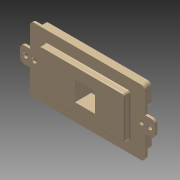
# Autodesk Inventor part: Wall_Switch_June_8_2017_Front._Sppt
Saved by Autodesk Inventor 2015 (Build 190159000, 159)
## iProperties
Created: 2014-05-05
Part Number: Wall_Switch_June_8_2017_Front._Sppt
Material: ABS Plastic
Document SubType Name: Modeling
Designer: admin
Density: 1.06 g/cm^3
Appearance: Smooth - Off-White
Author: admin
Autodesk Inventor part; units mm, degrees
sketch "Sketch1" plane through (0, 0, 0) normal (0, 0, 1) x (1, 0, 0)
  line L0 (-46.99, 28.575) -> (46.99, 28.575)
  line L1 (46.99, 28.575) -> (46.99, -28.575)
  line L2 (46.99, -28.575) -> (-46.99, -28.575)
  line L3 (-46.99, -28.575) -> (-46.99, 28.575)
  line L4 (45.2735, 26.416) -> (-44.3885, 26.416)
  line L5 (-44.831, -26.416) -> (44.831, -26.416)
  circle A0 centre (41.656, 0) radius 1.5875
  circle A1 centre (-41.656, -0.0059) radius 1.5875
  arc A2 (41.656, 3.175) -> (41.656, -3.175) centre (41.656, 0) ccw
  line L6 (-41.656, 3.1691) -> (-44.3885, 3.1691)
  line L7 (-41.656, -3.1809) -> (-44.831, -3.1809)
  line L8 (41.656, -3.175) -> (44.831, -3.175)
  line L9 (41.656, 3.175) -> (45.2735, 3.175)
  line L10 (44.831, -26.416) -> (44.831, -3.175)
  line L11 (45.2735, 3.175) -> (45.2735, 26.416)
  line L12 (-44.3885, 26.416) -> (-44.3885, 3.1691)
  arc A3 (-41.656, -3.1809) -> (-41.656, 3.1691) centre (-41.656, -0.0059) ccw
  line L13 (-44.831, -3.1809) -> (-44.831, -26.416)
  point P0 (0, 0)
  point P1 (0, 28.575)
  point P2 (-46.99, 0)
  constraints: 28 end point, 11 perpendicular, 7 parallel, 4 centre point, 4 point on circle, 4 tangent, 2 midpoint, 1 horizontal, 1 horizontal alignment, 1 vertical alignment
ref_plane "Work Plane1" through (0, 0, 0) normal (0, 0, 1) x (1, 0, 0)
sketch "Sketch2" plane through (0, 0, 0) normal (0, 0, 1) x (1, 0, 0)
  circle A0 centre (-41.656, -0.0059) radius 1.5875 projected
  circle A1 centre (41.656, 0) radius 1.5875 projected
  line L0 (-52.451, 25.4) -> (52.451, 25.4)
  line L1 (52.451, 25.4) -> (52.451, -25.4)
  line L2 (52.451, -25.4) -> (-52.451, -25.4)
  line L3 (-52.451, -25.4) -> (-52.451, 25.4)
  circle A2 centre (-41.656, -0.0059) radius 1.5875
  circle A3 centre (41.656, 0) radius 1.5875
  point P0 (0, 0)
  point P1 (0, 25.4)
  point P2 (52.451, 0)
  point P3 (-41.656, 0)
  point P4 (0, 12.7)
  dimension "d10" = 104.902
  dimension "d11" = 50.8
  constraints: 8 end point, 2 centre point, 2 coincident, 2 horizontal alignment, 2 midpoint, 2 parallel, 2 vertical alignment, 1 horizontal, 1 perpendicular
  measures "d10" distance of L1.end L2.end
  measures "d11" distance of L0.end L1.end
extrude "Extrusion2" add sketch "Sketch2" along normal blind 1.905
ref_plane "Work Plane3" through (0, 0, 2.54) normal (0, 0, 1) x (1, 0, 0)
sketch "Sketch4" plane through (0, 0, 2.54) normal (0, 0, 1) x (1, 0, 0)
  line L0 (-33.0835, 16.383) -> (33.0835, 16.383)
  line L1 (33.0835, 16.383) -> (33.0835, -16.383)
  line L2 (33.0835, -16.383) -> (-33.0835, -16.383)
  line L3 (-33.0835, -16.383) -> (-33.0835, 16.383)
  point P0 (0, 0)
  point P1 (0, 16.383)
  point P2 (33.0835, 0)
  dimension "d22" = 66.167
  dimension "d23" = 32.766
  constraints: 8 end point, 2 midpoint, 2 parallel, 1 horizontal, 1 horizontal alignment, 1 perpendicular, 1 vertical alignment
  measures "d22" distance of L1.end L2.end
  measures "d23" distance of L0.end L1.end
ref_plane "Work Plane2" through (0, 0, 0) normal (0, 0, -1) x (-1, 0, 0)
sketch "Sketch5" plane through (0, 0, 0) normal (0, 0, -1) x (-1, 0, 0)
  line L0 (44.3885, 3.1691) -> (44.3885, 25.4) projected
  line L1 (-45.2735, 25.4) -> (-45.2735, 3.175) projected
  line L2 (-45.2735, 3.175) -> (-41.656, 3.175) projected
  arc A0 (-41.656, -3.175) -> (-41.656, 3.175) centre (-41.656, 0) ccw projected
  line L3 (-41.656, -3.175) -> (-44.831, -3.175) projected
  line L4 (-44.831, -3.175) -> (-44.831, -25.4) projected
  line L5 (44.831, -25.4) -> (44.831, -3.1809) projected
  line L6 (44.831, -3.1809) -> (41.656, -3.1809) projected
  arc A1 (41.656, 3.1691) -> (41.656, -3.1809) centre (41.656, -0.0059) ccw projected
  line L7 (41.656, 3.1691) -> (44.3885, 3.1691) projected
  circle A2 centre (39.116, 12.7) radius 1.27
  circle A3 centre (39.116, -12.7) radius 1.27
  circle A4 centre (-39.116, -12.7) radius 1.27
  circle A5 centre (-39.116, 12.7) radius 1.27
  line L8 (-35.56, 20.32) -> (35.56, 20.32)
  line L9 (35.56, 20.32) -> (35.56, -20.32)
  line L10 (35.56, -20.32) -> (-35.56, -20.32)
  line L11 (-35.56, -20.32) -> (-35.56, 20.32)
  line L12 (46.99, -28.575) -> (46.99, 28.575) projected
  line L13 (-46.99, 28.575) -> (-46.99, -28.575) projected
  line L14 (-41.656, 22.86) -> (41.656, 22.86)
  line L15 (41.656, -22.86) -> (-41.656, -22.86)
  line L16 (-37.6174, 5.6991) -> (-37.6174, -5.6991)
  line L17 (37.6174, 5.6933) -> (37.6174, -5.705)
  arc A6 (37.6174, -5.705) -> (41.656, -6.9909) centre (41.656, -0.0059) ccw
  arc A7 (41.656, 6.9791) -> (37.6174, 5.6933) centre (41.656, -0.0059) ccw
  line L18 (41.656, 22.86) -> (41.656, 6.9791)
  line L19 (41.656, -6.9909) -> (41.656, -22.86)
  arc A8 (-37.6174, 5.6991) -> (-41.656, 6.985) centre (-41.656, 0) ccw
  arc A9 (-41.656, -6.985) -> (-37.6174, -5.6991) centre (-41.656, 0) ccw
  line L20 (-41.656, -22.86) -> (-41.656, -6.985)
  line L21 (-41.656, 6.985) -> (-41.656, 22.86)
  point P0 (0, 0)
  point P1 (-38.1, 0)
  point P2 (-35.56, 0)
  point P3 (0, 20.32)
  point P4 (0, 12.7)
  point P5 (41.656, -0.0059)
  dimension "d30" = 2.54
  dimension "d31" = 2.54
  dimension "d32" = 2.54
  dimension "d33" = 2.54
  dimension "d36" = 71.12
  dimension "d37" = 40.64
  dimension "d91" = 83.312
  dimension "d92" = 45.72
  dimension "d95" = 2.0574
  dimension "d205" = 2.54
  constraints: 26 end point, 10 parallel, 8 centre point, 8 point on circle, 4 vertical alignment, 3 coincident, 3 perpendicular, 2 horizontal, 2 horizontal alignment, 2 midpoint, 1 point on line
  measures "d30" diameter of A2
  measures "d31" diameter of A3
  measures "d32" diameter of A4
  measures "d33" diameter of A5
  measures "d36" distance of L9.end L10.end
  measures "d37" distance of L8.end L9.end
  measures "d91" distance of L15.start L15.end
  measures "d92" distance of L14.end L15.start
  measures "d95" distance between parallel lines of L17 L9
  measures "d205" distance between parallel lines of L8 L14
extrude "Extrusion8" add sketch "Sketch5" along normal blind 6.35
sketch "Sketch10" plane through (0, 0, 0) normal (0, 0, -1) x (-1, 0, 0)
  point P0 (0, 0)
sketch "Sketch7" plane through (0, 0, 0) normal (0, 0, -1) x (-1, 0, 0)
  line L0 (-33.02, 16.51) -> (33.02, 16.51)
  line L1 (33.02, 16.51) -> (33.02, -16.51)
  line L2 (33.02, -16.51) -> (-33.02, -16.51)
  line L3 (-33.02, -16.51) -> (-33.02, 16.51)
  point P0 (0, 0)
  point P1 (0, 16.51)
  point P2 (-33.02, 0)
  dimension "d55" = 66.04
  dimension "d56" = 33.02
  constraints: 8 end point, 2 midpoint, 2 parallel, 1 horizontal, 1 horizontal alignment, 1 perpendicular, 1 vertical alignment
  measures "d55" distance of L1.end L2.end
  measures "d56" distance of L0.end L1.end
sketch "Sketch8" plane through (0, 0, 1.905) normal (0, 0, 1) x (1, 0, 0)
  circle A0 centre (41.656, 0) radius 1.5875 projected
  circle A1 centre (-41.656, -0.0059) radius 1.5875 projected
  circle A2 centre (41.656, 0) radius 1.905
  circle A3 centre (-41.656, -0.0059) radius 1.905
  circle A4 centre (-48.387, 0) radius 1.905
  circle A5 centre (48.387, 0) radius 1.905
  point P0 (0, 0)
  dimension "d68" = 3.81
  dimension "d69" = 3.81
  dimension "d72" = 3.81
  dimension "d73" = 6.731
  dimension "d74" = 3.81
  dimension "d75" = 6.731
  constraints: 4 centre point, 2 coincident
  measures "d68" diameter of A2
  measures "d69" diameter of A3
  measures "d72" diameter of A4
  measures "d73" distance of A1.centre A4.centre
  measures "d74" diameter of A5
  measures "d75" distance of A5.centre A0.centre
extrude "Extrusion6" cut sketch "Sketch8" against normal blind 5.08
sketch "Sketch9" plane through (0, 0, 1.905) normal (0, 0, 1) x (1, 0, 0)
  line L0 (-52.451, 25.4) -> (-44.831, 25.4)
  line L1 (-44.831, 25.4) -> (-44.831, 6.35)
  line L2 (-44.831, 6.35) -> (-52.451, 6.35)
  line L3 (-52.451, 6.35) -> (-52.451, 25.4)
  line L4 (52.451, 25.4) -> (44.831, 25.4)
  line L5 (44.831, 25.4) -> (44.831, 6.35)
  line L6 (44.831, 6.35) -> (52.451, 6.35)
  line L7 (52.451, 6.35) -> (52.451, 25.4)
  line L8 (52.451, -25.4) -> (44.831, -25.4)
  line L9 (44.831, -25.4) -> (44.831, -6.35)
  line L10 (44.831, -6.35) -> (52.451, -6.35)
  line L11 (52.451, -6.35) -> (52.451, -25.4)
  line L12 (-52.451, -25.4) -> (-44.831, -25.4)
  line L13 (-44.831, -25.4) -> (-44.831, -6.35)
  line L14 (-44.831, -6.35) -> (-52.451, -6.35)
  line L15 (-52.451, -6.35) -> (-52.451, -25.4)
  line L16 (52.451, -25.4) -> (52.451, 25.4) projected
  point P0 (0, 0)
  point P1 (52.451, 15.875)
  point P2 (52.451, 0)
  dimension "d76" = 7.62
  dimension "d77" = 19.05
  dimension "d80" = 7.62
  dimension "d81" = 19.05
  dimension "d82" = 7.62
  dimension "d83" = 19.05
  dimension "d117" = 19.05
  dimension "d149" = 7.62
  constraints: 32 end point, 8 parallel, 4 horizontal, 4 perpendicular, 2 midpoint, 1 vertical alignment
  measures "d76" distance of L1.end L2.end
  measures "d77" distance of L0.end L1.end
  measures "d80" distance of L9.end L10.end
  measures "d81" distance of L8.end L9.end
  measures "d82" distance of L14.end L13.end
  measures "d83" distance of L13.end L12.end
  measures "d117" distance between parallel lines of L6 L4
  measures "d149" distance between parallel lines of L7 L5
extrude "Extrusion7" cut sketch "Sketch9" against normal blind 5.08
fillet "Fillet5" radius 3.175 8 edges at (44.831, 25.4, 0.9525) (52.451, 6.35, 0.9525) (-44.831, 25.4, 0.9525) (-52.451, 6.35, 0.9525) (52.451, -6.35, 0.9525) (44.831, -25.4, 0.9525) (-44.831, -25.4, 0.9525) (-52.451, -6.35, 0.9525)
fillet "Fillet7" radius 3.175 4 edges at (-41.656, -22.86, -3.175) (-41.656, 22.86, -3.175) (41.656, 22.86, -3.175) (41.656, -22.86, -3.175)
fillet "Fillet8" radius 3.175 4 edges at (-41.656, 6.9791, -3.175) (-41.656, -6.9909, -3.175) (41.656, 6.985, -3.175) (41.656, -6.985, -3.175)
sketch "Sketch13" plane through (0, 0, -6.35) normal (0, 0, -1) x (-1, 0, 0)
  line L0 (37.6174, -5.705) -> (37.6174, 5.6933) projected
  arc A0 (39.4732, 6.6293) -> (37.6174, 5.6933) centre (41.656, -0.0059) ccw projected
  line L1 (-37.6174, 5.6991) -> (-37.6174, -5.6991) projected
  arc A1 (-39.4732, -6.6352) -> (-37.6174, -5.6991) centre (-41.656, 0) ccw projected
  arc A2 (-37.6174, -3.0816) -> (-37.6174, 3.0816) centre (-41.656, 0) ccw
  arc A3 (37.6174, 3.0757) -> (37.6174, -3.0874) centre (41.656, -0.0059) ccw
  line L2 (37.6174, -3.0874) -> (37.6174, 3.0757)
  line L3 (-37.6174, -3.0816) -> (-37.6174, 3.0816)
  point P0 (0, 0)
  dimension "d107" = 10.16
  dimension "d108" = 10.16
  constraints: 4 end point, 4 point on circle, 4 point on line, 2 centre point, 2 coincident, 2 collinear
  measures "d107" diameter of A2
  measures "d108" diameter of A3
extrude "Extrusion9" [suppressed]
fillet "Fillet11" [suppressed]
fillet "Fillet12" [suppressed]
extrude "Extrusion17" add sketch "Sketch7" against normal blind 6.35
sketch "Sketch22" plane through (0, 0, 0) normal (0, 0, -1) x (-1, 0, 0)
  line L0 (-10.16, -7.7495) -> (5.3391, -7.7495)
  line L1 (5.3391, -7.7495) -> (5.3391, 7.7495)
  line L2 (5.3391, 7.7495) -> (-10.16, 7.7495)
  line L3 (-10.16, 7.7495) -> (-10.16, -7.7495)
  line L4 (-33.02, 16.51) -> (-33.02, -16.51) projected
  line L5 (41.656, 9.6453) -> (41.656, 19.685) projected
  point P0 (0, 0)
  point P1 (-33.02, 15.875)
  point P2 (-33.02, -15.875)
  point P3 (-10.16, 0)
  dimension "d194" = 15.4991
  dimension "d195" = 15.4991
  dimension "d197" = 51.816
  constraints: 8 end point, 2 parallel, 1 horizontal, 1 horizontal alignment, 1 midpoint, 1 perpendicular
  measures "d194" distance of L2.end L0.start
  measures "d195" distance of L1.end L2.end
  measures "d197" distance between parallel lines of L3 L5
extrude "Extrusion18" cut sketch "Sketch22" against normal blind 25.4
sketch "Sketch23" plane through (0, 0, 0) normal (0, 0, -1) x (-1, 0, 0)
  line L0 (5.3391, 7.7495) -> (-10.16, 7.7495)
  line L1 (-10.16, 7.7495) -> (-10.16, -7.7495)
  line L2 (-10.16, -7.7495) -> (5.3391, -7.7495)
  line L3 (5.3391, -7.7495) -> (5.3391, 7.7495)
  line L4 (-11.684, 9.2735) -> (6.8631, 9.2735)
  line L5 (6.8631, 9.2735) -> (6.8631, -9.2735)
  line L6 (6.8631, -9.2735) -> (-11.684, -9.2735)
  line L7 (-11.684, -9.2735) -> (-11.684, 9.2735)
  point P0 (0, 0)
  dimension "d201" = 1.524
  constraints: 16 end point, 4 parallel, 2 perpendicular, 1 horizontal, 3 other
  measures "d201" distance between parallel lines of L0 L4
extrude "Extrusion19" add sketch "Sketch23" along normal blind 6.35
fillet "Fillet17" radius 1.27 4 edges at (11.684, 9.2735, -3.175) (-6.8631, 9.2735, -3.175) (11.684, -9.2735, -3.175) (-6.8631, -9.2735, -3.175)
fillet "Fillet20" radius 1.905 4 edges at (-33.02, -16.51, 4.1275) (-33.02, 16.51, 4.1275) (33.02, -16.51, 4.1275) (33.02, 16.51, 4.1275)
sketch "Sketch24" plane through (0, 0, -6.35) normal (0, 0, -1) x (-1, 0, 0)
  circle A0 centre (37.5285, 18.7325) radius 1.5875
  line L0 (-35.56, 20.32) -> (35.56, 20.32)
  line L1 (35.56, 20.32) -> (35.56, -20.32)
  line L2 (35.56, -20.32) -> (-35.56, -20.32)
  line L3 (-35.56, -20.32) -> (-35.56, 20.32)
  line L4 (35.56, -20.32) -> (35.56, 20.32) projected
  line L5 (38.0025, 17.2174) -> (43.4689, 17.2174) construction
  line L6 (41.656, 9.6453) -> (41.656, 19.685) projected
  line L7 (35.56, 20.32) -> (-35.56, 20.32) projected
  line L8 (35.56, 20.32) -> (37.5285, 20.32)
  line L9 (38.7245, 17.6886) -> (35.56, 13.335)
  circle A1 centre (37.5285, -18.7325) radius 1.5875
  line L10 (35.56, -20.32) -> (37.5285, -20.32)
  line L11 (35.56, -13.335) -> (38.9189, -17.9663)
  circle A2 centre (-37.5285, 18.7325) radius 1.5875
  line L12 (-41.656, 19.685) -> (-41.656, 9.6512) projected
  line L13 (-35.56, 20.32) -> (-37.5285, 20.32)
  line L14 (-35.56, -20.32) -> (-35.56, 20.32) projected
  line L15 (-38.7245, 17.6886) -> (-38.481, 17.4625)
  line L16 (-38.7245, 17.6886) -> (-35.56, 13.335)
  circle A3 centre (-37.5285, -18.7325) radius 1.5875
  line L17 (-35.56, -20.32) -> (-37.5285, -20.32)
  line L18 (-38.8115, -17.7977) -> (-35.56, -13.335)
  point P0 (0, 0)
  point P1 (35.56, 13.3804)
  dimension "d209" = 3.175
  dimension "d210" = 2.54
  dimension "d211" = 1.5875
  dimension "d212" = 3.175
  dimension "d213" = 1.5875
  dimension "d214" = 6.985
  dimension "d215" = 6.985
  dimension "d216" = 3.175
  dimension "d217" = 4.1275
  dimension "d218" = 3.175
  constraints: 28 end point, 11 point on circle, 5 horizontal alignment, 5 point on line, 4 centre point, 3 tangent, 2 horizontal, 2 parallel, 2 perpendicular, 2 vertical alignment, 1 collinear
  measures "d209" diameter of A0
  measures "d210" distance edge to line of A0 L6
  measures "d211" distance from line of A0.centre L0
  measures "d212" diameter of A1
  measures "d213" distance from line of L2 A1.centre
  measures "d214" distance of L9.end L0.end
  measures "d215" distance of L11.start L1.end
  measures "d216" diameter of A2
  measures "d217" distance from line of A2.centre L12
  measures "d218" diameter of A3
extrude "Extrusion20" cut sketch "Sketch24" against normal blind 6.35 contours A0 | A0 L9 L1 L8 | L3 L16 A2 L13 | L11 A1 L10 L1 | A2 L15 | L11 A1 | L3 L17 A3 L18 | A3 picked at (-37.2522, 18.6899) picked at (37.9734, -18.2759)
fillet "Fillet18" radius 3.175 4 edges at (35.56, 13.335, -3.175) (35.56, -13.335, -3.175) (-35.56, 13.335, -3.175) (-35.56, -13.335, -3.175)
fillet "Fillet21" radius 0.635 16 edges at (-32.462, -15.952, 6.35) (0, -16.51, 6.35) (32.462, -15.952, 6.35) (33.02, 0, 6.35) (32.462, 15.952, 6.35) (0, 16.51, 6.35) (-32.462, 15.952, 6.35) (-33.02, 0, 6.35) (-32.462, 15.952, 1.905) (0, 16.51, 1.905) (32.462, 15.952, 1.905) (33.02, 0, 1.905) (32.462, -15.952, 1.905) (0, -16.51, 1.905) (-32.462, -15.952, 1.905) (-33.02, 0, 1.905)
sketch "Sketch25" plane through (0, 0, 6.35) normal (0, 0, 1) x (1, 0, 0)
  line L0 (-44.831, 25.4) -> (44.8432, 25.4)
  line L1 (44.8432, 25.4) -> (44.8432, -25.4054)
  line L2 (44.8432, -25.4054) -> (-44.831, -25.4054)
  line L3 (-44.831, -25.4054) -> (-44.831, 25.4)
  line L4 (42.3032, -22.8654) -> (42.3032, 22.86)
  line L5 (42.3032, 22.86) -> (-42.291, 22.86)
  line L6 (-42.291, 22.86) -> (-42.291, -22.8654)
  line L7 (-42.291, -22.8654) -> (42.3032, -22.8654)
  line L8 (39.7632, 20.32) -> (39.7632, -20.3254)
  line L9 (39.7632, -20.3254) -> (-39.751, -20.3254)
  line L10 (-39.751, -20.3254) -> (-39.751, 20.32)
  line L11 (-39.751, 20.32) -> (39.7632, 20.32)
  line L12 (37.2232, -17.7854) -> (37.2232, 17.78)
  line L13 (37.2232, 17.78) -> (-37.211, 17.78)
  line L14 (-37.211, 17.78) -> (-37.211, -17.7854)
  line L15 (-37.211, -17.7854) -> (37.2232, -17.7854)
  point P0 (0, 0)
  dimension "d220" = 2.54
  dimension "d221" = 2.54
  dimension "d222" = 2.54
  constraints: 32 end point, 8 parallel, 4 perpendicular, 1 horizontal, 9 other
  measures "d220" distance between parallel lines of L1 L4
  measures "d221" distance between parallel lines of L4 L8
  measures "d222" distance between parallel lines of L8 L12
extrude "Extrusion21" [suppressed]
sketch "Sketch26" plane through (0, 0, 4.445) normal (0, 0, -1) x (-1, 0, 0)
  line L0 (-44.8432, -25.4054) -> (44.831, -25.4054)
  line L1 (44.831, -25.4054) -> (44.831, 25.4)
  line L2 (44.831, 25.4) -> (-44.8432, 25.4)
  line L3 (-44.8432, 25.4) -> (-44.8432, -25.4054)
  point P0 (0, 0)
  constraints: 8 end point, 2 parallel, 1 horizontal, 1 perpendicular
extrude "Extrusion22" [suppressed]
sketch "Sketch27" plane through (0, 0, 4.445) normal (0, 0, -1) x (-1, 0, 0)
  circle A0 centre (-43.5732, -24.1354) radius 0.635
  line L0 (-44.8432, 25.4) -> (-44.8432, -25.4054) projected
  line L1 (-44.8432, -25.4054) -> (44.831, -25.4054) projected
  circle A1 centre (-43.5732, 24.1246) radius 0.635
  circle A2 centre (-38.4424, -24.1354) radius 0.635
  circle A3 centre (-38.4424, 24.1246) radius 0.635
  circle A4 centre (-33.3116, -24.1354) radius 0.635
  circle A5 centre (-33.3116, 24.1246) radius 0.635
  circle A6 centre (-28.1808, -24.1354) radius 0.635
  circle A7 centre (-28.1808, 24.1246) radius 0.635
  circle A8 centre (-23.05, -24.1354) radius 0.635
  circle A9 centre (-23.05, 24.1246) radius 0.635
  circle A10 centre (-17.9192, -24.1354) radius 0.635
  circle A11 centre (-17.9192, 24.1246) radius 0.635
  circle A12 centre (-12.7884, -24.1354) radius 0.635
  circle A13 centre (-12.7884, 24.1246) radius 0.635
  circle A14 centre (-7.6576, -24.1354) radius 0.635
  circle A15 centre (-7.6576, 24.1246) radius 0.635
  circle A16 centre (-2.5268, -24.1354) radius 0.635
  circle A17 centre (-2.5268, 24.1246) radius 0.635
  circle A18 centre (2.604, -24.1354) radius 0.635
  circle A19 centre (2.604, 24.1246) radius 0.635
  circle A20 centre (7.7348, -24.1354) radius 0.635
  circle A21 centre (7.7348, 24.1246) radius 0.635
  circle A22 centre (12.8656, -24.1354) radius 0.635
  circle A23 centre (12.8656, 24.1246) radius 0.635
  circle A24 centre (17.9964, -24.1354) radius 0.635
  circle A25 centre (17.9964, 24.1246) radius 0.635
  circle A26 centre (23.1272, -24.1354) radius 0.635
  circle A27 centre (23.1272, 24.1246) radius 0.635
  circle A28 centre (28.258, -24.1354) radius 0.635
  circle A29 centre (28.258, 24.1246) radius 0.635
  circle A30 centre (33.3888, -24.1354) radius 0.635
  circle A31 centre (33.3888, 24.1246) radius 0.635
  circle A32 centre (38.5196, -24.1354) radius 0.635
  circle A33 centre (38.5196, 24.1246) radius 0.635
  circle A34 centre (43.6504, -24.1354) radius 0.635
  circle A35 centre (43.6504, 24.1246) radius 0.635
  circle A36 centre (-39.0774, -19.6078) radius 0.635
  circle A37 centre (-33.8958, -19.6078) radius 0.635
  circle A38 centre (-28.7142, -19.6078) radius 0.635
  circle A39 centre (-23.5326, -19.6078) radius 0.635
  circle A40 centre (-18.351, -19.6078) radius 0.635
  circle A41 centre (-13.1694, -19.6078) radius 0.635
  circle A42 centre (-7.9878, -19.6078) radius 0.635
  circle A43 centre (-2.8062, -19.6078) radius 0.635
  circle A44 centre (2.3754, -19.6078) radius 0.635
  circle A45 centre (7.557, -19.6078) radius 0.635
  circle A46 centre (12.7386, -19.6078) radius 0.635
  circle A47 centre (17.9202, -19.6078) radius 0.635
  circle A48 centre (23.1018, -19.6078) radius 0.635
  circle A49 centre (28.2834, -19.6078) radius 0.635
  circle A50 centre (33.465, -19.6078) radius 0.635
  circle A51 centre (38.6466, -19.6078) radius 0.635
  circle A52 centre (-39.0774, 19.2542) radius 0.635
  circle A53 centre (-33.8958, 19.2542) radius 0.635
  circle A54 centre (-28.7142, 19.2542) radius 0.635
  circle A55 centre (-23.5326, 19.2542) radius 0.635
  circle A56 centre (-18.351, 19.2542) radius 0.635
  circle A57 centre (-13.1694, 19.2542) radius 0.635
  circle A58 centre (-7.9878, 19.2542) radius 0.635
  circle A59 centre (-2.8062, 19.2542) radius 0.635
  circle A60 centre (2.3754, 19.2542) radius 0.635
  circle A61 centre (7.557, 19.2542) radius 0.635
  circle A62 centre (12.7386, 19.2542) radius 0.635
  circle A63 centre (17.9202, 19.2542) radius 0.635
  circle A64 centre (23.1018, 19.2542) radius 0.635
  circle A65 centre (28.2834, 19.2542) radius 0.635
  circle A66 centre (33.465, 19.2542) radius 0.635
  circle A67 centre (38.6466, 19.2542) radius 0.635
  point P0 (0, 0)
  dimension "d227" = 1.27
  dimension "d228" = 1.27
  dimension "d229" = 1.27
  dimension "d232" = 48.26
  dimension "d235" = 5.1308
  dimension "d238" = 1.27
  dimension "d241" = 5.1816
  dimension "d244" = 38.862
  constraints: 68 centre point, 2 horizontal, 2 vertical, 132 other
  measures "d227" diameter of A0
  measures "d228" distance from line of L0 A0.centre
  measures "d229" distance from line of L1 A0.centre
  measures "d232" distance of A0.centre A1.centre
  measures "d235" distance of A0.centre A2.centre
  measures "d238" diameter of A36
  measures "d241" distance of A36.centre A37.centre
  measures "d244" distance of A36.centre A52.centre
extrude "Extrusion23" [suppressed]
sketch "Sketch28" plane through (0, 0, 4.445) normal (0, 0, -1) x (-1, 0, 0)
  circle A0 centre (-43.6894, 20.8151) radius 0.635
  line L0 (44.831, 25.0594) -> (-44.8432, 25.0594)
  line L1 (-44.8432, 25.0594) -> (-44.8432, -26.0034)
  circle A1 centre (-43.6894, 15.7351) radius 0.635
  circle A2 centre (-43.6894, 10.6551) radius 0.635
  circle A3 centre (-43.6894, 5.5751) radius 0.635
  circle A4 centre (-43.6894, 0.4951) radius 0.635
  circle A5 centre (-43.6894, -4.5849) radius 0.635
  circle A6 centre (-43.6894, -9.6649) radius 0.635
  circle A7 centre (-43.6894, -14.7449) radius 0.635
  circle A8 centre (-43.6894, -19.8249) radius 0.635
  circle A9 centre (43.6866, 20.8151) radius 0.635
  circle A10 centre (43.6866, 15.7351) radius 0.635
  circle A11 centre (43.6866, 10.6551) radius 0.635
  circle A12 centre (43.6866, 5.5751) radius 0.635
  circle A13 centre (43.6866, 0.4951) radius 0.635
  circle A14 centre (43.6866, -4.5849) radius 0.635
  circle A15 centre (43.6866, -9.6649) radius 0.635
  circle A16 centre (43.6866, -14.7449) radius 0.635
  circle A17 centre (43.6866, -19.8249) radius 0.635
  circle A18 centre (-38.6023, 15.7351) radius 0.508
  circle A19 centre (-38.6023, 10.6551) radius 0.508
  circle A20 centre (-38.6023, 5.5751) radius 0.508
  circle A21 centre (-38.6023, 0.4951) radius 0.508
  circle A22 centre (-38.6023, -4.5849) radius 0.508
  circle A23 centre (-38.6023, -9.6649) radius 0.508
  circle A24 centre (-38.6023, -14.7449) radius 0.508
  circle A25 centre (38.8677, 15.7351) radius 0.508
  circle A26 centre (38.8677, 10.6551) radius 0.508
  circle A27 centre (38.8677, 5.5751) radius 0.508
  circle A28 centre (38.8677, 0.4951) radius 0.508
  circle A29 centre (38.8677, -4.5849) radius 0.508
  circle A30 centre (38.8677, -9.6649) radius 0.508
  circle A31 centre (38.8677, -14.7449) radius 0.508
  point P0 (0, 0)
  dimension "d249" = 1.27
  dimension "d252" = 5.08
  dimension "d255" = 87.376
  dimension "d258" = 1.016
  dimension "d261" = 5.08
  dimension "d264" = 77.47
  constraints: 32 centre point, 4 end point, 2 horizontal, 2 vertical, 60 other
  measures "d249" diameter of A0
  measures "d252" distance of A0.centre A1.centre
  measures "d255" distance of A0.centre A9.centre
  measures "d258" diameter of A18
  measures "d261" distance of A18.centre A19.centre
  measures "d264" distance of A18.centre A25.centre
extrude "Extrusion24" [suppressed]
sketch "Sketch30" plane through (0, 0, 6.35) normal (0, 0, 1) x (1, 0, 0)
  circle A0 centre (-49.9255, -4.769) radius 0.508
  arc A1 (33.02, 15.875) -> (32.385, 16.51) centre (32.385, 15.875) ccw projected
  line L0 (-39.751, -20.3254) -> (32.834, -20.3254)
  line L1 (32.834, -20.3254) -> (32.834, 16.324)
  circle A2 centre (49.1345, -4.769) radius 0.508
  circle A3 centre (-49.9255, 4.629) radius 0.508
  circle A4 centre (49.1345, 4.629) radius 0.508
  point P0 (0, 0)
  dimension "d269" = 1.016
  dimension "d272" = 99.06
  dimension "d275" = 9.398
  constraints: 4 centre point, 4 end point, 2 horizontal, 1 perpendicular, 1 point on circle, 1 vertical, 6 other
  measures "d269" diameter of A0
  measures "d272" distance of A0.centre A2.centre
  measures "d275" distance of A0.centre A3.centre
extrude "Extrusion25" [suppressed]
sketch "Sketch31" plane through (0, 0, 6.35) normal (0, 0, 1) x (1, 0, 0)
  line L0 (-51.3775, -6.3094) -> (-48.8375, -6.3094)
  line L1 (-48.8375, -6.3094) -> (-48.8375, 6.3906)
  line L2 (-48.8375, 6.3906) -> (-51.3775, 6.3906)
  line L3 (-51.3775, 6.3906) -> (-51.3775, -6.3094)
  line L4 (50.8969, -6.3094) -> (48.3569, -6.3094)
  line L5 (48.3569, -6.3094) -> (48.3569, 6.3906)
  line L6 (48.3569, 6.3906) -> (50.8969, 6.3906)
  line L7 (50.8969, 6.3906) -> (50.8969, -6.3094)
  point P0 (0, 0)
  dimension "d280" = 2.54
  dimension "d281" = 12.7
  dimension "d282" = 2.54
  constraints: 16 end point, 4 parallel, 2 horizontal, 2 perpendicular
  measures "d280" distance of L2.end L1.end
  measures "d281" distance of L1.end L0.end
  measures "d282" distance of L5.end L6.end
extrude "Extrusion26" [suppressed]
fillet "Fillet19" [suppressed]
body "Solid1"
